Autodesk Fusion 360 part; units mm, degrees
note: some values were not read from the file. Chosen so that the rebuilt part matches the saved one: a direction. Set by a fixed rule: which sketch regions a step uses.
(part 6 of 8)
  spline S38 degree 5 poles (-19.283, -48.8907) (-19.2856, -48.8958) (-19.2906, -48.9059) (-19.2978, -48.9213) (-19.3066, -48.9421) (-19.3166, -48.9686) (-19.3259, -48.9954) (-19.3347, -49.0225) (-19.3433, -49.0496) (-19.3517, -49.0768) (-19.36, -49.1042) (-19.368, -49.1316) (-19.3757, -49.1592) (-19.3831, -49.1869) (-19.3902, -49.2147) (-19.3969, -49.2427) (-19.4033, -49.2709) (-19.4094, -49.2991) (-19.4154, -49.3274) (-19.4211, -49.3558) (-19.4267, -49.3843) (-19.4321, -49.4128) (-19.4372, -49.4415) (-19.4421, -49.4702) (-19.4468, -49.4991) (-19.4513, -49.528) (-19.4556, -49.557) (-19.4597, -49.586) (-19.4636, -49.6152) (-19.4673, -49.6444) (-19.4708, -49.6737) (-19.4741, -49.703) (-19.4773, -49.7324) (-19.4803, -49.7619) (-19.4831, -49.7914) (-19.4857, -49.821) (-19.4881, -49.8507) (-19.4904, -49.8804) (-19.4925, -49.9102) (-19.4944, -49.94) (-19.4962, -49.9699) (-19.4978, -49.9999) (-19.4992, -50.0299) (-19.5004, -50.0599) (-19.5015, -50.09) (-19.5025, -50.1202) (-19.5033, -50.1504) (-19.5039, -50.1807) (-19.5043, -50.211) (-19.5046, -50.2413) (-19.5048, -50.2717) (-19.5048, -50.3022) (-19.5046, -50.3326) (-19.5043, -50.3632) (-19.5038, -50.3938) (-19.5032, -50.4244) (-19.5025, -50.455) (-19.5015, -50.4857) (-19.5005, -50.5165) (-19.4993, -50.5472) (-19.4979, -50.5781) (-19.4964, -50.6089) (-19.4947, -50.6398) (-19.4929, -50.6707) (-19.491, -50.7017) (-19.4889, -50.7327) (-19.4867, -50.7637) (-19.4843, -50.7948) (-19.4818, -50.8259) (-19.4791, -50.857) (-19.4764, -50.8882) (-19.474, -50.9131) (-19.4722, -50.9319) (-19.4709, -50.9444) (-19.4703, -50.9506) knots 0 0 0 0 0 0 0.01428571 0.02857143 0.04285714 0.05714286 0.07142857 0.08571429 0.1 0.11428571 0.12857143 0.14285714 0.15714286 0.17142857 0.18571429 0.2 0.21428571 0.22857143 0.24285714 0.25714286 0.27142857 0.28571429 0.3 0.31428571 0.32857143 0.34285714 0.35714286 0.37142857 0.38571429 0.4 0.41428571 0.42857143 0.44285714 0.45714286 0.47142857 0.48571429 0.5 0.51428571 0.52857143 0.54285714 0.55714286 0.57142857 0.58571429 0.6 0.61428571 0.62857143 0.64285714 0.65714286 0.67142857 0.68571429 0.7 0.71428571 0.72857143 0.74285714 0.75714286 0.77142857 0.78571429 0.8 0.81428571 0.82857143 0.84285714 0.85714286 0.87142857 0.88571429 0.9 0.91428571 0.92857143 0.94285714 0.95714286 0.97142857 0.98571429 1 1 1 1 1 1
  arc A78 (-19.4703, -50.9506) -> (-18.7268, -51.2588) centre (-13.5, -37.5997) ccw
  spline S39 degree 5 poles (-18.7268, -51.2588) (-18.7219, -51.2549) (-18.7122, -51.2469) (-18.6976, -51.235) (-18.6783, -51.219) (-18.6543, -51.1989) (-18.6304, -51.1788) (-18.6066, -51.1586) (-18.583, -51.1384) (-18.5594, -51.118) (-18.536, -51.0976) (-18.5128, -51.0771) (-18.4896, -51.0565) (-18.4666, -51.0358) (-18.4437, -51.0151) (-18.4209, -50.9943) (-18.3983, -50.9734) (-18.3758, -50.9524) (-18.3534, -50.9314) (-18.3312, -50.9102) (-18.3091, -50.889) (-18.2871, -50.8678) (-18.2653, -50.8464) (-18.2436, -50.825) (-18.2221, -50.8035) (-18.2007, -50.7819) (-18.1794, -50.7602) (-18.1583, -50.7385) (-18.1373, -50.7166) (-18.1165, -50.6947) (-18.0958, -50.6728) (-18.0753, -50.6507) (-18.0549, -50.6286) (-18.0347, -50.6064) (-18.0147, -50.5841) (-17.9947, -50.5617) (-17.975, -50.5393) (-17.9554, -50.5167) (-17.936, -50.4941) (-17.9167, -50.4714) (-17.8976, -50.4487) (-17.8787, -50.4258) (-17.8599, -50.4029) (-17.8414, -50.3799) (-17.823, -50.3568) (-17.8047, -50.3336) (-17.7867, -50.3103) (-17.7688, -50.287) (-17.7511, -50.2636) (-17.7337, -50.24) (-17.7164, -50.2164) (-17.6993, -50.1927) (-17.6824, -50.1689) (-17.6658, -50.1451) (-17.6494, -50.1211) (-17.6332, -50.097) (-17.6171, -50.0729) (-17.6013, -50.0486) (-17.5857, -50.0243) (-17.5703, -49.9999) (-17.5553, -49.9754) (-17.5405, -49.9507) (-17.5261, -49.9259) (-17.5121, -49.901) (-17.4984, -49.8759) (-17.4849, -49.8508) (-17.4715, -49.8256) (-17.4584, -49.8003) (-17.4455, -49.7749) (-17.4331, -49.7494) (-17.4214, -49.7236) (-17.4129, -49.7027) (-17.4071, -49.6867) (-17.4035, -49.676) (-17.4017, -49.6706) knots -1 -1 -1 -1 -1 -1 -0.98571429 -0.97142857 -0.95714286 -0.94285714 -0.92857143 -0.91428571 -0.9 -0.88571429 -0.87142857 -0.85714286 -0.84285714 -0.82857143 -0.81428571 -0.8 -0.78571429 -0.77142857 -0.75714286 -0.74285714 -0.72857143 -0.71428571 -0.7 -0.68571429 -0.67142857 -0.65714286 -0.64285714 -0.62857143 -0.61428571 -0.6 -0.58571429 -0.57142857 -0.55714286 -0.54285714 -0.52857143 -0.51428571 -0.5 -0.48571429 -0.47142857 -0.45714286 -0.44285714 -0.42857143 -0.41428571 -0.4 -0.38571429 -0.37142857 -0.35714286 -0.34285714 -0.32857143 -0.31428571 -0.3 -0.28571429 -0.27142857 -0.25714286 -0.24285714 -0.22857143 -0.21428571 -0.2 -0.18571429 -0.17142857 -0.15714286 -0.14285714 -0.12857143 -0.11428571 -0.1 -0.08571429 -0.07142857 -0.05714286 -0.04285714 -0.02857143 -0.01428571 0 0 0 0 0 0
  line L39 (-17.4017, -49.6706) -> (-17.2824, -49.3016)
  arc A79 (-17.1573, -49.2369) -> (-17.2824, -49.3016) centre (-17.1873, -49.3323) ccw
  arc A80 (-17.1573, -49.2369) -> (-16.1582, -49.5049) centre (-13.5, -37.5997) ccw
  arc A81 (-16.0822, -49.6235) -> (-16.1582, -49.5049) centre (-16.18, -49.6025) ccw
  line L40 (-16.0822, -49.6235) -> (-16.1636, -50.0028)
  spline S40 degree 5 poles (-16.1636, -50.0028) (-16.1648, -50.0083) (-16.1671, -50.0194) (-16.17, -50.0361) (-16.1731, -50.0585) (-16.1759, -50.0867) (-16.178, -50.115) (-16.1795, -50.1434) (-16.1807, -50.1718) (-16.1818, -50.2003) (-16.1827, -50.2288) (-16.1834, -50.2574) (-16.1837, -50.286) (-16.1837, -50.3147) (-16.1833, -50.3434) (-16.1825, -50.3722) (-16.1814, -50.4011) (-16.18, -50.4299) (-16.1785, -50.4588) (-16.1767, -50.4877) (-16.1747, -50.5167) (-16.1725, -50.5457) (-16.17, -50.5747) (-16.1674, -50.6037) (-16.1644, -50.6328) (-16.1613, -50.6618) (-16.1579, -50.691) (-16.1543, -50.7201) (-16.1505, -50.7492) (-16.1466, -50.7784) (-16.1424, -50.8076) (-16.138, -50.8368) (-16.1335, -50.866) (-16.1287, -50.8953) (-16.1238, -50.9245) (-16.1186, -50.9538) (-16.1133, -50.9831) (-16.1078, -51.0124) (-16.1021, -51.0417) (-16.0962, -51.071) (-16.0902, -51.1003) (-16.084, -51.1297) (-16.0776, -51.159) (-16.071, -51.1884) (-16.0643, -51.2178) (-16.0574, -51.2471) (-16.0503, -51.2765) (-16.0431, -51.3059) (-16.0357, -51.3353) (-16.0281, -51.3647) (-16.0204, -51.3941) (-16.0125, -51.4235) (-16.0045, -51.4529) (-15.9963, -51.4823) (-15.9879, -51.5117) (-15.9794, -51.5411) (-15.9707, -51.5705) (-15.9619, -51.6) (-15.9529, -51.6294) (-15.9438, -51.6588) (-15.9345, -51.6882) (-15.925, -51.7176) (-15.9154, -51.747) (-15.9057, -51.7764) (-15.8958, -51.8058) (-15.8858, -51.8352) (-15.8756, -51.8646) (-15.8653, -51.894) (-15.8548, -51.9234) (-15.8442, -51.9528) (-15.8334, -51.9822) (-15.8247, -52.0057) (-15.8181, -52.0233) (-15.8136, -52.035) (-15.8114, -52.0409) knots 0 0 0 0 0 0 0.01428571 0.02857143 0.04285714 0.05714286 0.07142857 0.08571429 0.1 0.11428571 0.12857143 0.14285714 0.15714286 0.17142857 0.18571429 0.2 0.21428571 0.22857143 0.24285714 0.25714286 0.27142857 0.28571429 0.3 0.31428571 0.32857143 0.34285714 0.35714286 0.37142857 0.38571429 0.4 0.41428571 0.42857143 0.44285714 0.45714286 0.47142857 0.48571429 0.5 0.51428571 0.52857143 0.54285714 0.55714286 0.57142857 0.58571429 0.6 0.61428571 0.62857143 0.64285714 0.65714286 0.67142857 0.68571429 0.7 0.71428571 0.72857143 0.74285714 0.75714286 0.77142857 0.78571429 0.8 0.81428571 0.82857143 0.84285714 0.85714286 0.87142857 0.88571429 0.9 0.91428571 0.92857143 0.94285714 0.95714286 0.97142857 0.98571429 1 1 1 1 1 1
  arc A82 (-15.8114, -52.0409) -> (-15.0134, -52.1462) centre (-13.5, -37.5997) ccw
  spline S41 degree 5 poles (-15.0134, -52.1462) (-15.0098, -52.1411) (-15.0024, -52.1309) (-14.9915, -52.1156) (-14.977, -52.0952) (-14.9589, -52.0696) (-14.9411, -52.044) (-14.9233, -52.0183) (-14.9057, -51.9926) (-14.8883, -51.9669) (-14.8709, -51.9411) (-14.8538, -51.9152) (-14.8367, -51.8894) (-14.8198, -51.8634) (-14.8031, -51.8375) (-14.7865, -51.8115) (-14.77, -51.7854) (-14.7537, -51.7594) (-14.7376, -51.7333) (-14.7216, -51.7071) (-14.7057, -51.6809) (-14.69, -51.6547) (-14.6744, -51.6284) (-14.659, -51.6021) (-14.6438, -51.5757) (-14.6287, -51.5493) (-14.6138, -51.5229) (-14.599, -51.4964) (-14.5844, -51.4699) (-14.57, -51.4434) (-14.5557, -51.4168) (-14.5416, -51.3902) (-14.5276, -51.3635) (-14.5138, -51.3369) (-14.5002, -51.3101) (-14.4868, -51.2834) (-14.4735, -51.2566) (-14.4604, -51.2297) (-14.4475, -51.2029) (-14.4348, -51.176) (-14.4222, -51.149) (-14.4098, -51.1221) (-14.3977, -51.0951) (-14.3857, -51.068) (-14.3739, -51.041) (-14.3623, -51.0138) (-14.3509, -50.9867) (-14.3397, -50.9595) (-14.3287, -50.9323) (-14.3178, -50.9051) (-14.3073, -50.8778) (-14.2969, -50.8505) (-14.2868, -50.8232) (-14.2769, -50.7958) (-14.2672, -50.7684) (-14.2578, -50.7409) (-14.2486, -50.7135) (-14.2396, -50.686) (-14.2308, -50.6584) (-14.2222, -50.6309) (-14.214, -50.6033) (-14.2062, -50.5756) (-14.1987, -50.548) (-14.1916, -50.5202) (-14.1848, -50.4925) (-14.1783, -50.4647) (-14.1719, -50.4369) (-14.1658, -50.4091) (-14.1599, -50.3812) (-14.1545, -50.3534) (-14.1499, -50.3254) (-14.1471, -50.303) (-14.1456, -50.2861) (-14.1449, -50.2748) (-14.1446, -50.2692) knots -1 -1 -1 -1 -1 -1 -0.98571429 -0.97142857 -0.95714286 -0.94285714 -0.92857143 -0.91428571 -0.9 -0.88571429 -0.87142857 -0.85714286 -0.84285714 -0.82857143 -0.81428571 -0.8 -0.78571429 -0.77142857 -0.75714286 -0.74285714 -0.72857143 -0.71428571 -0.7 -0.68571429 -0.67142857 -0.65714286 -0.64285714 -0.62857143 -0.61428571 -0.6 -0.58571429 -0.57142857 -0.55714286 -0.54285714 -0.52857143 -0.51428571 -0.5 -0.48571429 -0.47142857 -0.45714286 -0.44285714 -0.42857143 -0.41428571 -0.4 -0.38571429 -0.37142857 -0.35714286 -0.34285714 -0.32857143 -0.31428571 -0.3 -0.28571429 -0.27142857 -0.25714286 -0.24285714 -0.22857143 -0.21428571 -0.2 -0.18571429 -0.17142857 -0.15714286 -0.14285714 -0.12857143 -0.11428571 -0.1 -0.08571429 -0.07142857 -0.05714286 -0.04285714 -0.02857143 -0.01428571 0 0 0 0 0 0
  line L41 (-14.1446, -50.2692) -> (-14.1249, -49.8818)
  arc A83 (-14.0208, -49.787) -> (-14.1249, -49.8818) centre (-14.025, -49.8869) ccw
  arc A84 (-14.0208, -49.787) -> (-12.9863, -49.7873) centre (-13.5, -37.5997) ccw
  arc A85 (-12.8822, -49.8822) -> (-12.9863, -49.7873) centre (-12.9821, -49.8872) ccw
  line L42 (-12.8822, -49.8822) -> (-12.8627, -50.2695)
  spline S42 degree 5 poles (-12.8627, -50.2695) (-12.8624, -50.2752) (-12.8617, -50.2865) (-12.8603, -50.3034) (-12.8575, -50.3258) (-12.8529, -50.3538) (-12.8475, -50.3816) (-12.8416, -50.4095) (-12.8355, -50.4373) (-12.8292, -50.4651) (-12.8227, -50.4929) (-12.8159, -50.5206) (-12.8088, -50.5484) (-12.8014, -50.576) (-12.7935, -50.6037) (-12.7853, -50.6313) (-12.7768, -50.6589) (-12.768, -50.6864) (-12.759, -50.7139) (-12.7498, -50.7414) (-12.7404, -50.7688) (-12.7308, -50.7962) (-12.7209, -50.8236) (-12.7108, -50.851) (-12.7004, -50.8783) (-12.6899, -50.9056) (-12.6791, -50.9328) (-12.6681, -50.96) (-12.6569, -50.9872) (-12.6455, -51.0143) (-12.6339, -51.0415) (-12.6221, -51.0685) (-12.6102, -51.0956) (-12.598, -51.1226) (-12.5856, -51.1496) (-12.5731, -51.1765) (-12.5604, -51.2034) (-12.5475, -51.2303) (-12.5344, -51.2571) (-12.5211, -51.2839) (-12.5077, -51.3107) (-12.4941, -51.3374) (-12.4804, -51.3641) (-12.4664, -51.3908) (-12.4523, -51.4174) (-12.4381, -51.444) (-12.4236, -51.4706) (-12.409, -51.4971) (-12.3943, -51.5235) (-12.3794, -51.55) (-12.3643, -51.5764) (-12.3491, -51.6027) (-12.3337, -51.6291) (-12.3181, -51.6553) (-12.3025, -51.6816) (-12.2866, -51.7078) (-12.2706, -51.734) (-12.2545, -51.7601) (-12.2382, -51.7862) (-12.2217, -51.8122) (-12.2052, -51.8382) (-12.1884, -51.8642) (-12.1716, -51.8901) (-12.1545, -51.916) (-12.1374, -51.9419) (-12.1201, -51.9677) (-12.1026, -51.9934) (-12.085, -52.0191) (-12.0673, -52.0448) (-12.0494, -52.0704) (-12.0314, -52.096) (-12.0169, -52.1165) (-12.006, -52.1318) (-11.9987, -52.142) (-11.995, -52.1471) knots 0 0 0 0 0 0 0.01428571 0.02857143 0.04285714 0.05714286 0.07142857 0.08571429 0.1 0.11428571 0.12857143 0.14285714 0.15714286 0.17142857 0.18571429 0.2 0.21428571 0.22857143 0.24285714 0.25714286 0.27142857 0.28571429 0.3 0.31428571 0.32857143 0.34285714 0.35714286 0.37142857 0.38571429 0.4 0.41428571 0.42857143 0.44285714 0.45714286 0.47142857 0.48571429 0.5 0.51428571 0.52857143 0.54285714 0.55714286 0.57142857 0.58571429 0.6 0.61428571 0.62857143 0.64285714 0.65714286 0.67142857 0.68571429 0.7 0.71428571 0.72857143 0.74285714 0.75714286 0.77142857 0.78571429 0.8 0.81428571 0.82857143 0.84285714 0.85714286 0.87142857 0.88571429 0.9 0.91428571 0.92857143 0.94285714 0.95714286 0.97142857 0.98571429 1 1 1 1 1 1
  arc A86 (-11.995, -52.1471) -> (-11.197, -52.0422) centre (-13.5, -37.5997) ccw
  spline S43 degree 5 poles (-11.197, -52.0422) (-11.1947, -52.0364) (-11.1903, -52.0246) (-11.1837, -52.007) (-11.1749, -51.9835) (-11.1641, -51.9542) (-11.1535, -51.9248) (-11.143, -51.8954) (-11.1327, -51.866) (-11.1225, -51.8366) (-11.1124, -51.8072) (-11.1025, -51.7778) (-11.0928, -51.7484) (-11.0831, -51.719) (-11.0737, -51.6896) (-11.0644, -51.6602) (-11.0552, -51.6308) (-11.0462, -51.6014) (-11.0374, -51.572) (-11.0287, -51.5426) (-11.0201, -51.5132) (-11.0118, -51.4837) (-11.0035, -51.4543) (-10.9955, -51.4249) (-10.9876, -51.3955) (-10.9798, -51.3661) (-10.9723, -51.3367) (-10.9648, -51.3074) (-10.9576, -51.278) (-10.9505, -51.2486) (-10.9436, -51.2192) (-10.9368, -51.1899) (-10.9303, -51.1605) (-10.9239, -51.1312) (-10.9176, -51.1018) (-10.9116, -51.0725) (-10.9057, -51.0432) (-10.9, -51.0139) (-10.8945, -50.9846) (-10.8891, -50.9553) (-10.884, -50.926) (-10.879, -50.8968) (-10.8742, -50.8676) (-10.8697, -50.8383) (-10.8653, -50.8091) (-10.8611, -50.7799) (-10.8571, -50.7508) (-10.8533, -50.7216) (-10.8497, -50.6925) (-10.8463, -50.6634) (-10.8431, -50.6343) (-10.8402, -50.6052) (-10.8375, -50.5762) (-10.835, -50.5472) (-10.8328, -50.5182) (-10.8308, -50.4893) (-10.829, -50.4604) (-10.8274, -50.4315) (-10.826, -50.4026) (-10.8249, -50.3738) (-10.8241, -50.345) (-10.8237, -50.3163) (-10.8236, -50.2876) (-10.8239, -50.259) (-10.8246, -50.2304) (-10.8255, -50.2019) (-10.8265, -50.1734) (-10.8278, -50.1449) (-10.8293, -50.1165) (-10.8313, -50.0882) (-10.8341, -50.06) (-10.8372, -50.0376) (-10.8401, -50.0209) (-10.8424, -50.0098) (-10.8435, -50.0043) knots -1 -1 -1 -1 -1 -1 -0.98571429 -0.97142857 -0.95714286 -0.94285714 -0.92857143 -0.91428571 -0.9 -0.88571429 -0.87142857 -0.85714286 -0.84285714 -0.82857143 -0.81428571 -0.8 -0.78571429 -0.77142857 -0.75714286 -0.74285714 -0.72857143 -0.71428571 -0.7 -0.68571429 -0.67142857 -0.65714286 -0.64285714 -0.62857143 -0.61428571 -0.6 -0.58571429 -0.57142857 -0.55714286 -0.54285714 -0.52857143 -0.51428571 -0.5 -0.48571429 -0.47142857 -0.45714286 -0.44285714 -0.42857143 -0.41428571 -0.4 -0.38571429 -0.37142857 -0.35714286 -0.34285714 -0.32857143 -0.31428571 -0.3 -0.28571429 -0.27142857 -0.25714286 -0.24285714 -0.22857143 -0.21428571 -0.2 -0.18571429 -0.17142857 -0.15714286 -0.14285714 -0.12857143 -0.11428571 -0.1 -0.08571429 -0.07142857 -0.05714286 -0.04285714 -0.02857143 -0.01428571 0 0 0 0 0 0
  line L43 (-10.8435, -50.0043) -> (-10.9248, -49.625)
  arc A87 (-10.8487, -49.5065) -> (-10.9248, -49.625) centre (-10.827, -49.6041) ccw
  arc A88 (-10.8487, -49.5065) -> (-9.8494, -49.239) centre (-13.5, -37.5997) ccw
  arc A89 (-9.7243, -49.3037) -> (-9.8494, -49.239) centre (-9.8195, -49.3345) ccw
  line L44 (-9.7243, -49.3037) -> (-9.6053, -49.6729)
  spline S44 degree 5 poles (-9.6053, -49.6729) (-9.6035, -49.6783) (-9.5999, -49.689) (-9.5941, -49.7049) (-9.5856, -49.7259) (-9.574, -49.7517) (-9.5616, -49.7772) (-9.5487, -49.8026) (-9.5355, -49.8279) (-9.5222, -49.8531) (-9.5088, -49.8782) (-9.495, -49.9033) (-9.481, -49.9282) (-9.4666, -49.9531) (-9.4519, -49.9777) (-9.4368, -50.0023) (-9.4215, -50.0267) (-9.4059, -50.051) (-9.3901, -50.0753) (-9.3741, -50.0994) (-9.3579, -50.1235) (-9.3415, -50.1475) (-9.3248, -50.1714) (-9.308, -50.1952) (-9.2909, -50.2189) (-9.2737, -50.2425) (-9.2562, -50.266) (-9.2385, -50.2895) (-9.2207, -50.3128) (-9.2026, -50.3361) (-9.1844, -50.3593) (-9.166, -50.3824) (-9.1475, -50.4054) (-9.1287, -50.4284) (-9.1098, -50.4512) (-9.0907, -50.474) (-9.0715, -50.4967) (-9.0521, -50.5193) (-9.0325, -50.5419) (-9.0128, -50.5643) (-8.9929, -50.5867) (-8.9728, -50.609) (-8.9526, -50.6312) (-8.9323, -50.6534) (-8.9117, -50.6754) (-8.8911, -50.6974) (-8.8703, -50.7193) (-8.8493, -50.7412) (-8.8282, -50.7629) (-8.807, -50.7846) (-8.7856, -50.8062) (-8.764, -50.8277) (-8.7424, -50.8492) (-8.7206, -50.8705) (-8.6986, -50.8918) (-8.6765, -50.913) (-8.6543, -50.9342) (-8.6319, -50.9552) (-8.6095, -50.9762) (-8.5868, -50.9971) (-8.5641, -51.0179) (-8.5412, -51.0387) (-8.5182, -51.0594) (-8.495, -51.08) (-8.4718, -51.1005) (-8.4484, -51.1209) (-8.4249, -51.1413) (-8.4012, -51.1616) (-8.3775, -51.1818) (-8.3536, -51.2019) (-8.3296, -51.222) (-8.3103, -51.238) (-8.2957, -51.2499) (-8.286, -51.2579) (-8.2811, -51.2619) knots 0 0 0 0 0 0 0.01428571 0.02857143 0.04285714 0.05714286 0.07142857 0.08571429 0.1 0.11428571 0.12857143 0.14285714 0.15714286 0.17142857 0.18571429 0.2 0.21428571 0.22857143 0.24285714 0.25714286 0.27142857 0.28571429 0.3 0.31428571 0.32857143 0.34285714 0.35714286 0.37142857 0.38571429 0.4 0.41428571 0.42857143 0.44285714 0.45714286 0.47142857 0.48571429 0.5 0.51428571 0.52857143 0.54285714 0.55714286 0.57142857 0.58571429 0.6 0.61428571 0.62857143 0.64285714 0.65714286 0.67142857 0.68571429 0.7 0.71428571 0.72857143 0.74285714 0.75714286 0.77142857 0.78571429 0.8 0.81428571 0.82857143 0.84285714 0.85714286 0.87142857 0.88571429 0.9 0.91428571 0.92857143 0.94285714 0.95714286 0.97142857 0.98571429 1 1 1 1 1 1
  arc A90 (-8.2811, -51.2619) -> (-7.5374, -50.9541) centre (-13.5, -37.5997) ccw
  spline S45 degree 5 poles (-7.5374, -50.9541) (-7.5368, -50.9478) (-7.5355, -50.9353) (-7.5337, -50.9166) (-7.5313, -50.8916) (-7.5285, -50.8605) (-7.5259, -50.8293) (-7.5233, -50.7982) (-7.5209, -50.7672) (-7.5187, -50.7362) (-7.5166, -50.7052) (-7.5146, -50.6742) (-7.5128, -50.6433) (-7.5112, -50.6124) (-7.5096, -50.5815) (-7.5082, -50.5507) (-7.507, -50.5199) (-7.5059, -50.4892) (-7.505, -50.4585) (-7.5042, -50.4278) (-7.5036, -50.3972) (-7.5031, -50.3667) (-7.5028, -50.3361) (-7.5026, -50.3056) (-7.5026, -50.2752) (-7.5027, -50.2448) (-7.503, -50.2144) (-7.5034, -50.1841) (-7.504, -50.1539) (-7.5048, -50.1237) (-7.5057, -50.0935) (-7.5068, -50.0634) (-7.508, -50.0333) (-7.5094, -50.0033) (-7.511, -49.9734) (-7.5127, -49.9435) (-7.5147, -49.9137) (-7.5167, -49.8839) (-7.519, -49.8542) (-7.5214, -49.8245) (-7.524, -49.7949) (-7.5268, -49.7653) (-7.5297, -49.7359) (-7.5329, -49.7065) (-7.5362, -49.6771) (-7.5397, -49.6478) (-7.5434, -49.6186) (-7.5473, -49.5895) (-7.5513, -49.5604) (-7.5556, -49.5314) (-7.5601, -49.5025) (-7.5647, -49.4737) (-7.5696, -49.4449) (-7.5748, -49.4163) (-7.5801, -49.3877) (-7.5857, -49.3592) (-7.5914, -49.3308) (-7.5974, -49.3025) (-7.6035, -49.2743) (-7.6099, -49.2461) (-7.6166, -49.2181) (-7.6236, -49.1903) (-7.631, -49.1626) (-7.6387, -49.135) (-7.6467, -49.1076) (-7.6549, -49.0802) (-7.6633, -49.053) (-7.6719, -49.0258) (-7.6807, -48.9988) (-7.69, -48.972) (-7.7, -48.9455) (-7.7088, -48.9246) (-7.7159, -48.9093) (-7.7209, -48.8991) (-7.7235, -48.8941) knots -1 -1 -1 -1 -1 -1 -0.98571429 -0.97142857 -0.95714286 -0.94285714 -0.92857143 -0.91428571 -0.9 -0.88571429 -0.87142857 -0.85714286 -0.84285714 -0.82857143 -0.81428571 -0.8 -0.78571429 -0.77142857 -0.75714286 -0.74285714 -0.72857143 -0.71428571 -0.7 -0.68571429 -0.67142857 -0.65714286 -0.64285714 -0.62857143 -0.61428571 -0.6 -0.58571429 -0.57142857 -0.55714286 -0.54285714 -0.52857143 -0.51428571 -0.5 -0.48571429 -0.47142857 -0.45714286 -0.44285714 -0.42857143 -0.41428571 -0.4 -0.38571429 -0.37142857 -0.35714286 -0.34285714 -0.32857143 -0.31428571 -0.3 -0.28571429 -0.27142857 -0.25714286 -0.24285714 -0.22857143 -0.21428571 -0.2 -0.18571429 -0.17142857 -0.15714286 -0.14285714 -0.12857143 -0.11428571 -0.1 -0.08571429 -0.07142857 -0.05714286 -0.04285714 -0.02857143 -0.01428571 0 0 0 0 0 0
  line L45 (-7.7235, -48.8941) -> (-7.9001, -48.5488)
  arc A91 (-7.8574, -48.4146) -> (-7.9001, -48.5488) centre (-7.8111, -48.5032) ccw
  arc A92 (-7.8574, -48.4146) -> (-6.9613, -47.8976) centre (-13.5, -37.5997) ccw
  arc A93 (-6.8238, -47.9277) -> (-6.9613, -47.8976) centre (-6.9077, -47.982) ccw
  line L46 (-6.8238, -47.9277) -> (-6.6132, -48.2535)
  spline S46 degree 5 poles (-6.6132, -48.2535) (-6.6101, -48.2582) (-6.6039, -48.2677) (-6.5941, -48.2815) (-6.5805, -48.2996) (-6.5626, -48.3215) (-6.544, -48.3429) (-6.525, -48.3641) (-6.5058, -48.3851) (-6.4864, -48.406) (-6.4668, -48.4268) (-6.4471, -48.4475) (-6.4271, -48.468) (-6.4068, -48.4882) (-6.3862, -48.5082) (-6.3653, -48.528) (-6.3441, -48.5477) (-6.3228, -48.5671) (-6.3012, -48.5864) (-6.2795, -48.6056) (-6.2576, -48.6247) (-6.2356, -48.6436) (-6.2133, -48.6624) (-6.1909, -48.681) (-6.1683, -48.6995) (-6.1455, -48.7178) (-6.1225, -48.736) (-6.0994, -48.7541) (-6.0761, -48.772) (-6.0527, -48.7899) (-6.0291, -48.8076) (-6.0053, -48.8251) (-5.9814, -48.8426) (-5.9574, -48.8599) (-5.9332, -48.8771) (-5.9089, -48.8941) (-5.8844, -48.9111) (-5.8598, -48.9279) (-5.8351, -48.9446) (-5.8102, -48.9612) (-5.7852, -48.9776) (-5.76, -48.994) (-5.7348, -49.0102) (-5.7094, -49.0264) (-5.6838, -49.0424) (-5.6582, -49.0583) (-5.6324, -49.074) (-5.6065, -49.0897) (-5.5805, -49.1052) (-5.5544, -49.1207) (-5.5281, -49.136) (-5.5017, -49.1512) (-5.4753, -49.1663) (-5.4487, -49.1813) (-5.422, -49.1962) (-5.3951, -49.211) (-5.3682, -49.2256) (-5.3412, -49.2402) (-5.314, -49.2546) (-5.2867, -49.269) (-5.2594, -49.2832) (-5.2319, -49.2973) (-5.2043, -49.3114) (-5.1766, -49.3253) (-5.1489, -49.3391) (-5.121, -49.3528) (-5.093, -49.3663) (-5.0649, -49.3798) (-5.0367, -49.3932) (-5.0084, -49.4065) (-4.98, -49.4196) (-4.9572, -49.4301) (-4.9401, -49.4378) (-4.9287, -49.443) (-4.9229, -49.4456) knots 0 0 0 0 0 0 0.01428571 0.02857143 0.04285714 0.05714286 0.07142857 0.08571429 0.1 0.11428571 0.12857143 0.14285714 0.15714286 0.17142857 0.18571429 0.2 0.21428571 0.22857143 0.24285714 0.25714286 0.27142857 0.28571429 0.3 0.31428571 0.32857143 0.34285714 0.35714286 0.37142857 0.38571429 0.4 0.41428571 0.42857143 0.44285714 0.45714286 0.47142857 0.48571429 0.5 0.51428571 0.52857143 0.54285714 0.55714286 0.57142857 0.58571429 0.6 0.61428571 0.62857143 0.64285714 0.65714286 0.67142857 0.68571429 0.7 0.71428571 0.72857143 0.74285714 0.75714286 0.77142857 0.78571429 0.8 0.81428571 0.82857143 0.84285714 0.85714286 0.87142857 0.88571429 0.9 0.91428571 0.92857143 0.94285714 0.95714286 0.97142857 0.98571429 1 1 1 1 1 1
  arc A94 (-4.9229, -49.4456) -> (-4.2842, -48.9558) centre (-13.5, -37.5997) ccw
  spline S47 degree 5 poles (-4.2842, -48.9558) (-4.2852, -48.9496) (-4.2873, -48.9372) (-4.2903, -48.9186) (-4.2945, -48.8939) (-4.2999, -48.8631) (-4.3053, -48.8323) (-4.311, -48.8016) (-4.3167, -48.771) (-4.3225, -48.7405) (-4.3285, -48.71) (-4.3347, -48.6796) (-4.3409, -48.6492) (-4.3473, -48.619) (-4.3538, -48.5888) (-4.3604, -48.5586) (-4.3672, -48.5286) (-4.3741, -48.4986) (-4.3812, -48.4687) (-4.3884, -48.4389) (-4.3957, -48.4092) (-4.4031, -48.3795) (-4.4107, -48.3499) (-4.4184, -48.3204) (-4.4263, -48.291) (-4.4343, -48.2617) (-4.4424, -48.2325) (-4.4507, -48.2033) (-4.4591, -48.1742) (-4.4676, -48.1453) (-4.4763, -48.1164) (-4.4852, -48.0876) (-4.4941, -48.0588) (-4.5033, -48.0302) (-4.5125, -48.0017) (-4.522, -47.9733) (-4.5315, -47.945) (-4.5412, -47.9167) (-4.5511, -47.8886) (-4.5611, -47.8606) (-4.5713, -47.8326) (-4.5816, -47.8048) (-4.5921, -47.7771) (-4.6027, -47.7495) (-4.6135, -47.722) (-4.6245, -47.6947) (-4.6356, -47.6674) (-4.6469, -47.6403) (-4.6584, -47.6132) (-4.67, -47.5863) (-4.6818, -47.5596) (-4.6938, -47.5329) (-4.7059, -47.5064) (-4.7183, -47.4801) (-4.7309, -47.4539) (-4.7436, -47.4278) (-4.7565, -47.4019) (-4.7696, -47.376) (-4.7828, -47.3504) (-4.7963, -47.3248) (-4.81, -47.2995) (-4.824, -47.2744) (-4.8383, -47.2495) (-4.8528, -47.2249) (-4.8677, -47.2005) (-4.8827, -47.1762) (-4.8979, -47.1521) (-4.9132, -47.1281) (-4.9287, -47.1042) (-4.9446, -47.0807) (-4.9611, -47.0577) (-4.975, -47.0399) (-4.9859, -47.0269) (-4.9934, -47.0184) (-4.9971, -47.0142) knots -1 -1 -1 -1 -1 -1 -0.98571429 -0.97142857 -0.95714286 -0.94285714 -0.92857143 -0.91428571 -0.9 -0.88571429 -0.87142857 -0.85714286 -0.84285714 -0.82857143 -0.81428571 -0.8 -0.78571429 -0.77142857 -0.75714286 -0.74285714 -0.72857143 -0.71428571 -0.7 -0.68571429 -0.67142857 -0.65714286 -0.64285714 -0.62857143 -0.61428571 -0.6 -0.58571429 -0.57142857 -0.55714286 -0.54285714 -0.52857143 -0.51428571 -0.5 -0.48571429 -0.47142857 -0.45714286 -0.44285714 -0.42857143 -0.41428571 -0.4 -0.38571429 -0.37142857 -0.35714286 -0.34285714 -0.32857143 -0.31428571 -0.3 -0.28571429 -0.27142857 -0.25714286 -0.24285714 -0.22857143 -0.21428571 -0.2 -0.18571429 -0.17142857 -0.15714286 -0.14285714 -0.12857143 -0.11428571 -0.1 -0.08571429 -0.07142857 -0.05714286 -0.04285714 -0.02857143 -0.01428571 0 0 0 0 0 0
  line L47 (-4.9971, -47.0142) -> (-5.2571, -46.7263)
  arc A95 (-5.2505, -46.5856) -> (-5.2571, -46.7263) centre (-5.1829, -46.6593) ccw
  circle A96 centre (-13.5, -37.5997) radius 1.5
  line L48 (-17.5, -37.5997) -> (-17.5, -68.5997)
  arc A97 (-17.5, -68.5997) -> (-9.5, -68.5997) centre (-13.5, -68.5997) ccw
  line L49 (-9.5, -68.5997) -> (-9.5, -37.5997)
  arc A98 (-9.5, -37.5997) -> (-17.5, -37.5997) centre (-13.5, -37.5997) ccw
  line L50 (-13.5, -37.5997) -> (-13.5, -68.5997) construction
  circle A99 centre (-13.5, -68.5997) radius 1.5
  dimension "d70" = 31
  dimension "d71" = 4
  dimension "d72" = 3
  constraint tangent L48 A97
  constraint tangent A97 L49
  constraint parallel L48 L49
  constraint tangent L49 A98
  constraint tangent L48 A98
  constraint vertical L50
  constraint coincident A0.centre A2.centre
  constraint concentric A97 A99
  measures "d70" distance of A0.centre A97.centre
  measures "d71" radius of A97
  measures "d72" diameter of A99
extrude "Extrude3'" add sketch "Sketch6" against normal blind 3 contours S39 L39 A79 A80 A81 L40 S40 A82 S41 L41 A83 A84 A85 L42 S42 A86 S43 L43 A87 A88 A89 L44 S44 L48 A97 L49 | S39 L39 A79 A80 A81 L40 S40 A82 S41 L41 A83 A84 A85 L42 S42 A86 S43 L43 A87 A88 A89 L44 S44 L48 L49 A98 sketch seen with x (-0.793177, -0.608991, 0) y (0, 0, 1) z (-0.608991, 0.793177, 0) at (-12.19, 38.0446, -3) bodies 6 in component "Spur Gear 24 teeth (1)"
ref_plane "WorkPlane1" through (0, 1.5, -32.7497) normal (-1, 0, 0) x (0, 0, 1)
mirror "MirrorComponent1" about plane through (0, 0, 0) normal (0, 0, 1) of bodies 3 makes body 7 in component "Component2(Mirror)"
mirror "MirrorComponent1'" about plane through (0, 0, 0) normal (0, 0, 1) of bodies 2 makes body 8 in component "Component1(Mirror)"
sketch "Sketch7" plane through (0, 0, 0) normal (0, 0, 1) x (1, 0, 0)
  line L0 (55, 35) -> (55, 21)
  line L1 (55, 35) -> (52.5, 35)
  line L2 (52.5, 35) -> (52.5, 34)
  line L3 (52.5, 34) -> (53.5, 34)
  line L4 (53.5, 34) -> (53.5, 22)
  line L5 (53.5, 22) -> (52.5, 22)
  line L6 (52.5, 22) -> (52.5, 21)
  line L7 (52.5, 21) -> (55, 21)
  dimension "d127" = 14
  dimension "d128" = 1.5
  dimension "d129" = 2.5
  dimension "d130" = 1
  dimension "d131" = 1
  dimension "d132" = 2.5
  constraint vertical L0
  constraint perpendicular L0 L1
  constraint perpendicular L1 L2
  constraint perpendicular L2 L3
  constraint perpendicular L3 L4
  constraint perpendicular L4 L5
  constraint perpendicular L5 L6
  constraint horizontal L7
  measures "d127" distance of L0.start L0.end
  measures "d128" distance of L0 L4
  measures "d129" distance of L0 L2
  measures "d130" distance of L1.end L2.end
  measures "d131" distance of L5.end L6.end
  measures "d132" distance of L0 L6
revolve "Revolve1" add sketch "Sketch7" angle 360 about axis through (55, 35, 0) along (0, -1, 0) separate body makes body 9 in component "Component'''"
sketch "Base Circle (3)" plane through (0, 0, 0) normal (0, 0, 1) x (1, 0, 0) in component "Spur Gear 12 teeth"
  circle A0 centre (0, 0) radius 5.3273
  circle A1 centre (0, 0) radius 1.5
extrude "Extrude1'''''" add sketch "Base Circle (3)" along normal blind 6 separate body makes body 10 in component "Spur Gear 12 teeth"
sketch "Gear Tooth (3)" plane through (0, 0, 0) normal (0, 0, 1) x (1, 0, 0) in component "Spur Gear 12 teeth"
  spline S0 degree 5 poles (6.1362, -0.9011) (6.1405, -0.9017) (6.1493, -0.9029) (6.1624, -0.9042) (6.18, -0.9051) (6.202, -0.9052) (6.2242, -0.9045) (6.2464, -0.9033) (6.2686, -0.9019) (6.2909, -0.9002) (6.3132, -0.8984) (6.3355, -0.8963) (6.3578, -0.8939) (6.3802, -0.8912) (6.4026, -0.888) (6.425, -0.8845) (6.4474, -0.8806) (6.4699, -0.8765) (6.4923, -0.8722) (6.5148, -0.8676) (6.5373, -0.8629) (6.5598, -0.8579) (6.5822, -0.8526) (6.6047, -0.8471) (6.6272, -0.8414) (6.6497, -0.8354) (6.6722, -0.8292) (6.6947, -0.8228) (6.7172, -0.8162) (6.7397, -0.8093) (6.7622, -0.8023) (6.7847, -0.795) (6.8072, -0.7876) (6.8297, -0.7799) (6.8521, -0.7721) (6.8746, -0.764) (6.8971, -0.7558) (6.9195, -0.7474) (6.9419, -0.7387) (6.9644, -0.7299) (6.9868, -0.7209) (7.0092, -0.7117) (7.0315, -0.7023) (7.0539, -0.6928) (7.0763, -0.683) (7.0986, -0.6731) (7.1209, -0.663) (7.1432, -0.6527) (7.1655, -0.6423) (7.1877, -0.6317) (7.21, -0.6209) (7.2322, -0.6099) (7.2544, -0.5988) (7.2765, -0.5874) (7.2987, -0.576) (7.3208, -0.5643) (7.3429, -0.5525) (7.365, -0.5405) (7.387, -0.5284) (7.409, -0.516) (7.431, -0.5036) (7.453, -0.4909) (7.4749, -0.4781) (7.4968, -0.4652) (7.5187, -0.452) (7.5405, -0.4388) (7.5623, -0.4253) (7.5841, -0.4117) (7.6058, -0.398) (7.6275, -0.3841) (7.6492, -0.37) (7.6665, -0.3586) (7.6795, -0.35) (7.6881, -0.3443) (7.6924, -0.3414) knots 0 0 0 0 0 0 0.01428571 0.02857143 0.04285714 0.05714286 0.07142857 0.08571429 0.1 0.11428571 0.12857143 0.14285714 0.15714286 0.17142857 0.18571429 0.2 0.21428571 0.22857143 0.24285714 0.25714286 0.27142857 0.28571429 0.3 0.31428571 0.32857143 0.34285714 0.35714286 0.37142857 0.38571429 0.4 0.41428571 0.42857143 0.44285714 0.45714286 0.47142857 0.48571429 0.5 0.51428571 0.52857143 0.54285714 0.55714286 0.57142857 0.58571429 0.6 0.61428571 0.62857143 0.64285714 0.65714286 0.67142857 0.68571429 0.7 0.71428571 0.72857143 0.74285714 0.75714286 0.77142857 0.78571429 0.8 0.81428571 0.82857143 0.84285714 0.85714286 0.87142857 0.88571429 0.9 0.91428571 0.92857143 0.94285714 0.95714286 0.97142857 0.98571429 1 1 1 1 1 1
  spline S1 degree 5 poles (6.1362, 0.9011) (6.1405, 0.9017) (6.1493, 0.9029) (6.1624, 0.9042) (6.18, 0.9051) (6.202, 0.9052) (6.2242, 0.9045) (6.2464, 0.9033) (6.2686, 0.9019) (6.2909, 0.9002) (6.3132, 0.8984) (6.3355, 0.8963) (6.3578, 0.8939) (6.3802, 0.8912) (6.4026, 0.888) (6.425, 0.8845) (6.4474, 0.8806) (6.4699, 0.8765) (6.4923, 0.8722) (6.5148, 0.8676) (6.5373, 0.8629) (6.5598, 0.8579) (6.5822, 0.8526) (6.6047, 0.8471) (6.6272, 0.8414) (6.6497, 0.8354) (6.6722, 0.8292) (6.6947, 0.8228) (6.7172, 0.8162) (6.7397, 0.8093) (6.7622, 0.8023) (6.7847, 0.795) (6.8072, 0.7876) (6.8297, 0.7799) (6.8521, 0.7721) (6.8746, 0.764) (6.8971, 0.7558) (6.9195, 0.7474) (6.9419, 0.7387) (6.9644, 0.7299) (6.9868, 0.7209) (7.0092, 0.7117) (7.0315, 0.7023) (7.0539, 0.6928) (7.0763, 0.683) (7.0986, 0.6731) (7.1209, 0.663) (7.1432, 0.6527) (7.1655, 0.6423) (7.1877, 0.6317) (7.21, 0.6209) (7.2322, 0.6099) (7.2544, 0.5988) (7.2765, 0.5874) (7.2987, 0.576) (7.3208, 0.5643) (7.3429, 0.5525) (7.365, 0.5405) (7.387, 0.5284) (7.409, 0.516) (7.431, 0.5036) (7.453, 0.4909) (7.4749, 0.4781) (7.4968, 0.4652) (7.5187, 0.452) (7.5405, 0.4388) (7.5623, 0.4253) (7.5841, 0.4117) (7.6058, 0.398) (7.6275, 0.3841) (7.6492, 0.37) (7.6665, 0.3586) (7.6795, 0.35) (7.6881, 0.3443) (7.6924, 0.3414) knots 0 0 0 0 0 0 0.01428571 0.02857143 0.04285714 0.05714286 0.07142857 0.08571429 0.1 0.11428571 0.12857143 0.14285714 0.15714286 0.17142857 0.18571429 0.2 0.21428571 0.22857143 0.24285714 0.25714286 0.27142857 0.28571429 0.3 0.31428571 0.32857143 0.34285714 0.35714286 0.37142857 0.38571429 0.4 0.41428571 0.42857143 0.44285714 0.45714286 0.47142857 0.48571429 0.5 0.51428571 0.52857143 0.54285714 0.55714286 0.57142857 0.58571429 0.6 0.61428571 0.62857143 0.64285714 0.65714286 0.67142857 0.68571429 0.7 0.71428571 0.72857143 0.74285714 0.75714286 0.77142857 0.78571429 0.8 0.81428571 0.82857143 0.84285714 0.85714286 0.87142857 0.88571429 0.9 0.91428571 0.92857143 0.94285714 0.95714286 0.97142857 0.98571429 1 1 1 1 1 1
  arc A0 (7.6924, -0.3414) -> (7.6924, 0.3414) centre (0, 0) ccw
  line L0 (5.2609, -0.7725) -> (6.1362, -0.9011)
  line L1 (5.2609, 0.7725) -> (6.1362, 0.9011)
  line L2 (5.2609, -0.7725) -> (5.2609, 0.7725)
  point P0 (6.244, -0.9034)
  point P1 (6.3533, -0.8944)
  point P2 (6.4637, -0.8776)
  point P3 (6.5747, -0.8543)
  point P4 (6.6863, -0.8252)
  point P5 (6.7982, -0.7906)
  point P6 (6.9103, -0.7508)
  point P7 (7.0226, -0.7061)
  point P8 (7.1348, -0.6566)
  point P9 (7.247, -0.6024)
  point P10 (7.3589, -0.5438)
  point P11 (7.4705, -0.4806)
  point P12 (7.5817, -0.4132)
  point P13 (6.244, 0.9034)
  point P14 (6.3533, 0.8944)
  point P15 (6.4637, 0.8776)
  point P16 (6.5747, 0.8543)
  point P17 (6.6863, 0.8252)
  point P18 (6.7982, 0.7906)
  point P19 (6.9103, 0.7508)
  point P20 (7.0226, 0.7061)
  point P21 (7.1348, 0.6566)
  point P22 (7.247, 0.6024)
  point P23 (7.3589, 0.5438)
  point P24 (7.4705, 0.4806)
  point P25 (7.5817, 0.4132)
extrude "Extrude2'''" add sketch "Gear Tooth (3)" along normal blind 6 bodies 10 in component "Spur Gear 12 teeth"
fillet "Fillet1''" radius 0.1 2 edges at (5.2708, -0.774, 3) (5.2708, 0.774, 3) on bodies 10 in component "Spur Gear 12 teeth"
pattern_circular "C-Pattern1''" count 12 over 360 about axis through (0, 0, 0) along (0, 0, 1) of "Extrude2'''", "Fillet1''" in component "Spur Gear 12 teeth"
sketch "Diametrial Pitch Circle (3)" plane through (0, 0, 0) normal (0, 0, 1) x (1, 0, 0) in component "Spur Gear 12 teeth"
  circle A0 centre (0, 0) radius 6.6 construction